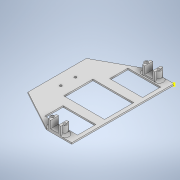
# Autodesk Inventor part: Part4
Saved by Autodesk Inventor 2020 (Build 240168000, 168)
## iProperties
Created: 2023-02-02
Part Number: Part4
Material: Generic
Document SubType Name: Modeling
Designer: aniela
Density: 1 g/cm^3
Appearance: Default
Author: aniela
Autodesk Inventor part; units mm, degrees
ref_plane "YZ Plane" through (0, 0, 0) normal (1, 0, 0) x (0, 1, 0)
ref_plane "XZ Plane" through (0, 0, 0) normal (0, 1, 0) x (-1, 0, 0)
ref_plane "XY Plane" through (0, 0, 0) normal (0, 0, 1) x (1, 0, 0)
sketch "Sketch1" plane through (0, 0, 0) normal (0, 1, 0) x (-1, 0, 0)
  line L0 (0, 0) -> (35, 0) construction
  line L1 (90, 30) -> (90, 110) construction
  line L2 (35, 140) -> (0, 140)
  line L3 (0, 140) -> (0, 0)
  line L4 (0, 0) -> (35, 0) construction
  line L5 (35, 0) -> (35, 140) construction
  line L6 (35, 140) -> (0, 140) construction
  line L7 (0, 140) -> (0, 0) construction
  line L8 (90, 110) -> (35, 140) construction
  line L9 (35, 0) -> (90, 30) construction
  line L10 (35, 140) -> (90, 110) construction
  line L11 (35, 0) -> (90, 30) construction
  line L12 (90, 110) -> (90, 30) construction
  line L13 (35, 0) -> (90, 30)
  line L14 (90, 30) -> (90, 110)
  line L15 (90, 110) -> (35, 140)
  line L16 (5, 127) -> (50, 127) construction
  line L17 (50, 127) -> (50, 102) construction
  line L18 (50, 102) -> (5, 102) construction
  line L19 (5, 102) -> (5, 127) construction
  line L20 (50, 127) -> (50, 102) construction
  line L21 (50, 102) -> (5, 102) construction
  line L22 (50, 127) -> (50, 102)
  line L23 (50, 127) -> (5, 127)
  line L24 (50, 102) -> (5, 102)
  line L25 (5, 102) -> (5, 127)
  line L26 (35, 0) -> (0, 0) construction
  line L27 (5, 13) -> (50, 13) construction
  line L28 (50, 13) -> (50, 38) construction
  line L29 (50, 38) -> (5, 38) construction
  line L30 (5, 38) -> (5, 13) construction
  line L31 (50, 38) -> (5, 38) construction
  line L32 (5, 38) -> (5, 13) construction
  line L33 (5, 13) -> (50, 13) construction
  line L34 (50, 13) -> (50, 38) construction
  line L35 (5, 13) -> (50, 13) construction
  line L36 (50, 13) -> (50, 38) construction
  line L37 (50, 38) -> (5, 38) construction
  line L38 (5, 38) -> (5, 13) construction
  line L39 (50, 38) -> (50, 13)
  line L40 (50, 13) -> (5, 13)
  line L41 (5, 13) -> (5, 38)
  line L42 (5, 38) -> (50, 38)
  line L43 (9.9818, 0) -> (0, 0) construction
  line L44 (0, 0) -> (0, 50) construction
  line L45 (0, 50) -> (9.9818, 50) construction
  line L46 (9.9818, 50) -> (9.9818, 0) construction
  line L47 (5, 50) -> (61, 50) construction
  line L48 (61, 50) -> (61, 87) construction
  line L49 (5, 87) -> (5, 50) construction
  line L50 (5, 87) -> (5, 50) construction
  line L51 (5, 50) -> (61, 50) construction
  line L52 (61, 50) -> (61, 87) construction
  line L53 (61, 87) -> (61, 50) construction
  line L54 (61, 50) -> (5, 50)
  line L55 (35, 0) -> (0, 0)
  line L56 (61, 50) -> (61, 90)
  line L57 (61, 90) -> (5, 90)
  line L58 (5, 50) -> (5, 90)
  point P0 (90, 140)
  point P1 (90, 0)
  dimension "d0" = 90
  dimension "d1" = 140
  dimension "d3" = 30
  dimension "d4" = 55
  dimension "d7" = 80
  dimension "d9" = 45
  dimension "d10" = 25
  dimension "d11" = 35
  dimension "d12" = 13
  dimension "d13" = 5
  dimension "d14" = 25
  dimension "d15" = 45
  dimension "d16" = 5
  dimension "d17" = 50
  dimension "d18" = 56
  dimension "d108" = 12
  dimension "d110" = 12
  dimension "d112" = 40
  constraints: 118 end point, 18 collinear, 16 parallel, 9 perpendicular, 9 point on line, 8 horizontal, 1 vertical
  measures "d0" distance of L2.end point (90, 140)
  measures "d1" distance of point (90, 140) point (90, 0)
  measures "d3" distance of L1.end point (90, 140)
  measures "d4" distance of L2.start point (90, 140)
  measures "d7" distance of L1.start L1.end
  measures "d9" distance of L17.end L18.end
  measures "d10" distance of L16.end L17.end
  measures "d11" distance of L2.start L2.end
  measures "d12" distance between parallel lines of L2 L16
  measures "d13" distance from line of L3 L18.end
  measures "d14" distance of L28.end L27.end
  measures "d15" distance of L28.end L31.end
  measures "d16" distance from line of L3 L27.start
  measures "d17" distance of L43.end L44.end
  measures "d18" distance of L49.start L48.end
  measures "d108" distance between parallel lines of L47 L37
  measures "d110" distance between parallel lines of L18 L57
  measures "d112" distance of L51.end L56.end
sketch "Sketch2" plane through (0, 0, 0) normal (0, 1, 0) x (-1, 0, 0)
  point P0 (0, 0)
sketch "Sketch3" plane through (0, 0, 0) normal (0, 1, 0) x (-1, 0, 0)
  point P0 (0, 0)
sketch "Sketch4" plane through (0, 0, 0) normal (0, 1, 0) x (-1, 0, 0)
  line L0 (0, 0) -> (35.5492, 0)
  line L1 (0, 0) -> (35, 0) construction
  line L2 (35, 0) -> (90, 30) construction
  line L3 (35, 0) -> (0, 0)
  constraints: 4 end point, 2 horizontal
extrude "Extrusion1" add sketch "Sketch1" along normal blind 2
sketch "Sketch5" plane through (0, 2, 0) normal (0, 1, 0) x (1, 0, 0)
  line L0 (0, 0) -> (-35, 0) projected
  line L1 (-15, 0) -> (-32, 0)
  line L2 (-32, 0) -> (-32, -11)
  line L3 (-32, -11) -> (-15, -11)
  line L4 (-15, -11) -> (-15, 0)
  line L5 (-32, 0) -> (-15, 0)
  line L6 (-15, 0) -> (-15, -11)
  line L7 (-15, -11) -> (-32, -11)
  line L8 (-32, -11) -> (-32, 0)
  line L9 (-35, -140) -> (0, -140) projected
  line L10 (-15, -140) -> (-32, -140)
  line L11 (-32, -140) -> (-32, -129)
  line L12 (-32, -129) -> (-15, -129)
  line L13 (-15, -129) -> (-15, -140)
  line L14 (-32, -129) -> (-15, -129)
  line L15 (-15, -129) -> (-15, -140)
  line L16 (-15, -140) -> (-32, -140)
  line L17 (-32, -140) -> (-32, -129)
  dimension "d22" = 17
  dimension "d23" = 11
  dimension "d24" = 11
  constraints: 32 end point, 8 parallel, 4 horizontal, 4 perpendicular, 4 point on line
  measures "d22" distance of L3.end L2.end
  measures "d23" distance of L2.end L1.end
  measures "d24" distance of L10.end L11.end
extrude "Extrusion2" add sketch "Sketch5" along normal blind 2
sketch "Sketch6" plane through (0, 4, 0) normal (0, 1, 0) x (1, 0, 0)
  line L0 (-32, 0) -> (-32, -11) projected
  line L1 (-32, 0) -> (-29, 0)
  line L2 (-29, 0) -> (-29, -11)
  line L3 (-29, -11) -> (-32, -11)
  line L4 (-32, -11) -> (-32, 0)
  line L5 (-15, -11) -> (-15, 0) projected
  line L6 (-32, -11) -> (-15, -11) projected
  line L7 (-15, 0) -> (-18, 0)
  line L8 (-18, 0) -> (-18, -11)
  line L9 (-18, -11) -> (-15, -11)
  line L10 (-15, -11) -> (-15, 0)
  line L11 (-32, -11) -> (-32, 0)
  line L12 (0, 0) -> (-35, 0) projected
  line L13 (-32, -11) -> (-15, -11)
  line L14 (-32, 0) -> (-15, 0)
  line L15 (-15, -129) -> (-15, -140) projected
  line L16 (-32, -129) -> (-15, -129) projected
  line L17 (-15, -140) -> (-18, -140)
  line L18 (-18, -140) -> (-18, -129)
  line L19 (-18, -129) -> (-15, -129)
  line L20 (-15, -129) -> (-15, -140)
  line L21 (-32, -129) -> (-29, -129)
  line L22 (-29, -129) -> (-29, -140)
  line L23 (-29, -140) -> (-32, -140)
  line L24 (-32, -140) -> (-32, -129)
  line L25 (-35, -140) -> (-32, -140) projected
  line L26 (-32, -140) -> (-32, -129)
  line L27 (-32, -129) -> (-15, -129)
  line L28 (-18, -129) -> (-18, -140)
  line L29 (-35, -140) -> (0, -140) projected
  line L30 (-29, -129) -> (-29, -140)
  dimension "d27" = 3
  dimension "d28" = 3
  constraints: 46 end point, 11 equal length, 8 perpendicular, 4 horizontal, 4 point on line
  measures "d27" distance of L2.end L3.end
  measures "d28" distance of L9.end L8.end
extrude "Extrusion3" add sketch "Sketch6" along normal blind 10 contours L15 L17 L18 L16 | L22 L23 L24 L16
sketch "Sketch7" plane through (0, 4, 0) normal (0, 1, 0) x (1, 0, 0)
  line L0 (-15, -11) -> (-15, 0) projected
  line L1 (-32, -11) -> (-15, -11) projected
  line L2 (-15, 0) -> (-18, 0)
  line L3 (-18, 0) -> (-18, -11)
  line L4 (-18, -11) -> (-15, -11)
  line L5 (-15, -11) -> (-15, 0)
  line L6 (-18, -11) -> (-15, -11)
  line L7 (-15, -11) -> (-15, 0)
  line L8 (-15, 0) -> (-18, 0)
  line L9 (-18, 0) -> (-18, -11)
  line L10 (-32, 0) -> (-32, -11) projected
  line L11 (-32, 0) -> (-29, 0)
  line L12 (-29, 0) -> (-29, -11)
  line L13 (-29, -11) -> (-32, -11)
  line L14 (-32, -11) -> (-32, 0)
  line L15 (-18, -11) -> (-29, -11)
  point P0 (0, 0)
  dimension "d31" = 3
  dimension "d32" = 3
  constraints: 26 end point, 6 parallel, 4 perpendicular, 3 horizontal, 2 point on line
  measures "d31" distance of L4.end L3.end
  measures "d32" distance of L12.end L13.end
extrude "Extrusion4" add sketch "Sketch7" along normal blind 10
sketch "Sketch8" plane through (0, 2, 0) normal (0, 1, 0) x (1, 0, 0)
  line L0 (-80, -55) -> (-70, -55)
  line L1 (-70, -55) -> (-70, -85)
  line L2 (-70, -85) -> (-80, -85)
  line L3 (-80, -85) -> (-80, -55)
  circle A0 centre (-75, -60) radius 1.5
  circle A1 centre (-75, -80) radius 1.5
  point P0 (0, 0)
  dimension "d35" = 10
  dimension "d36" = 30
  dimension "d37" = 3
  dimension "d38" = 3
  constraints: 8 end point, 2 centre point, 2 parallel, 1 horizontal, 1 perpendicular
  measures "d35" distance of L1.end L2.end
  measures "d36" distance of L0.end L1.end
  measures "d37" diameter of A0
  measures "d38" diameter of A1
extrude "Extrusion5" cut sketch "Sketch8" along normal blind 2
sketch "Sketch9" plane through (-75, 2, 80) normal (0, 1, 0) x (1, 0, 0)
  point P0 (75, 80)
  point P1 (-0.0687, 0.0063)
hole "Hole1" at (-75.0687, 2, 79.9937) direction (0, -1, 0) diameter 3 end through all
sketch "Sketch10" plane through (-75, 2, 60) normal (0, 1, 0) x (1, 0, 0)
  point P0 (75, 60)
  point P1 (-0.0342, 0.0658)
hole "Hole2" at (-75.0342, 2, 59.9342) direction (0, -1, 0) diameter 3 end through all
sketch "Sketch11" plane through (0, 14, 0) normal (0, 1, 0) x (1, 0, 0)
  line L0 (-15, 0) -> (-15, -11) projected
  circle A0 centre (-15, -5.5) radius 3
  line L1 (-32, -11) -> (-32, 0) projected
  circle A1 centre (-32, -5.5) radius 3
  point P0 (0, 0)
  point P1 (-15, -2.5)
  point P2 (-15, -8.5)
  point P3 (-32, -2.5)
  point P4 (-32, -8.5)
  dimension "d55" = 6
  dimension "d56" = 6
  constraints: 2 centre point, 2 midpoint
  measures "d55" diameter of A0
  measures "d56" diameter of A1
extrude "Extrusion6" add sketch "Sketch11" against normal blind 12 contours A0 L0 | A1 L1 picked at (-13.8765, -5.0912) picked at (-33.7524, -6.0681)
sketch "Sketch12" plane through (0, 14, 0) normal (0, 1, 0) x (1, 0, 0)
  arc A0 (-15, -8.5) -> (-15, -2.5) centre (-15, -5.5) ccw projected
  circle A1 centre (-15, -5.5) radius 2
  point P0 (0, 0)
  dimension "d59" = 4
  constraints: 1 centre point, 1 coincident
  measures "d59" diameter of A1
sketch "Sketch13" plane through (0, 14, 0) normal (0, 1, 0) x (1, 0, 0)
  arc A0 (-32, -2.5) -> (-32, -8.5) centre (-32, -5.5) ccw projected
  circle A1 centre (-32, -5.5) radius 2
  point P0 (0, 0)
  dimension "d60" = 4
  constraints: 1 centre point, 1 coincident
  measures "d60" diameter of A1
hole "Hole3" at (-32, 14, 5.5) direction (0, -1, 0) diameter 4 end through all
hole "Hole4" at (-15, 14, 5.5) direction (0, -1, 0) diameter 4 end through all
sketch "Sketch14" plane through (0, 0, 0) normal (0, -1, 0) x (1, 0, 0)
  circle A0 centre (-15, 5.5) radius 2 projected
  circle A1 centre (-15, 5.5) radius 2
  circle A2 centre (-32, 5.5) radius 2 projected
  circle A3 centre (-32, 5.5) radius 2
  circle A4 centre (-15, 5.5) radius 2
  point P0 (0, 0)
  constraints: 3 centre point, 3 coincident, 1 concentric
extrude "Extrusion7" add sketch "Sketch14" against normal blind 2
sketch "Sketch15" plane through (0, 14, 0) normal (0, 1, 0) x (1, 0, 0)
  line L0 (-15, -140) -> (-15, -129) projected
  circle A0 centre (-15, -134.5) radius 3
  line L1 (-18, -129) -> (-18, -140) projected
  point P0 (0, 0)
  constraints: 1 centre point, 1 midpoint, 1 tangent
extrude "Extrusion8" add sketch "Sketch15" against normal blind 12
sketch "Sketch16" plane through (0, 14, 0) normal (0, 1, 0) x (1, 0, 0)
  line L0 (-32, -140) -> (-32, -129) projected
  circle A0 centre (-32, -134.5) radius 3.0002
  point P0 (0, 0)
  point P1 (-32, -131.4998)
  point P2 (-32, -137.5002)
  constraints: 1 centre point, 1 midpoint
extrude "Extrusion9" add sketch "Sketch16" against normal blind 12 contours A0 L0 picked at (-33.3017, -133.9319)
sketch "Sketch17" plane through (0, 14, 0) normal (0, 1, 0) x (1, 0, 0)
  arc A0 (-15, -137.5) -> (-15, -131.5) centre (-15, -134.5) ccw projected
  circle A1 centre (-15, -134.5) radius 2
  arc A2 (-32, -131.4998) -> (-32, -137.5002) centre (-32, -134.5) ccw projected
  circle A3 centre (-32, -134.5) radius 2
  point P0 (0, 0)
  dimension "d81" = 4
  dimension "d82" = 4
  constraints: 2 centre point, 2 coincident
  measures "d81" diameter of A1
  measures "d82" diameter of A3
hole "Hole5" at (-32, 14, 134.5) direction (0, -1, 0) diameter 4 end through all
sketch "Sketch18" plane through (0, 14, 0) normal (0, 1, 0) x (1, 0, 0)
  arc A0 (-15, -137.5) -> (-15, -131.5) centre (-15, -134.5) ccw projected
  circle A1 centre (-15, -134.5) radius 2
  point P0 (0, 0)
  dimension "d7" = 80
  dimension "d11" = 35
  dimension "d90" = 4
  constraints: 1 centre point, 1 coincident
  measures "d90" diameter of A1
hole "Hole6" at (-15, 14, 134.5) direction (0, -1, 0) diameter 4 end through all
sketch "Sketch19" plane through (0, 0, 0) normal (0, -1, 0) x (1, 0, 0)
  point P0 (0, 0)
sketch "Sketch20" plane through (0, 14, 0) normal (0, 1, 0) x (1, 0, 0)
  circle A0 centre (-32, -134.5) radius 2 projected
  circle A1 centre (-32, -134.5) radius 2
  circle A2 centre (-15, -134.5) radius 2 projected
  circle A3 centre (-15, -134.5) radius 2
  point P0 (0, 0)
  constraints: 2 centre point, 2 coincident
extrude "Extrusion10" add sketch "Sketch20" against normal up to surface (14 mm away)
sketch "Sketch21" plane through (0, 0, 0) normal (0, -1, 0) x (1, 0, 0)
  point P0 (0, 0)
sketch "Sketch22" plane through (0, 14, 0) normal (0, 1, 0) x (1, 0, 0)
  arc A0 (-15, -137.5) -> (-15, -131.5) centre (-15, -134.5) ccw projected
  circle A1 centre (-15, -134.5) radius 2
  arc A2 (-32, -131.4998) -> (-32, -137.5002) centre (-32, -134.5) ccw projected
  circle A3 centre (-32, -134.5) radius 2
  point P0 (0, 0)
  dimension "d100" = 4
  dimension "d101" = 4
  constraints: 2 centre point, 2 coincident
  measures "d100" diameter of A1
  measures "d101" diameter of A3
extrude "Extrusion11" cut sketch "Sketch22" against normal blind 12 contours A1
sketch "Sketch23" plane through (0, 14, 0) normal (0, 1, 0) x (1, 0, 0)
  arc A0 (-32, -131.4998) -> (-32, -137.5002) centre (-32, -134.5) ccw projected
  circle A1 centre (-32, -134.5) radius 2
  point P0 (0, 0)
  dimension "d104" = 4
  constraints: 1 centre point, 1 coincident
  measures "d104" diameter of A1
extrude "Extrusion12" cut sketch "Sketch23" against normal blind 12
sketch "Sketch24" plane through (0, 2, 0) normal (0, 1, 0) x (1, 0, 0)
  point P0 (0, 0)
fillet "Fillet1" radius 3 1 edges at (-35, 2, 5.5)
fillet "Fillet2" radius 3 1 edges at (-12, 2, 5.5)
fillet "Fillet3" radius 3 1 edges at (-12, 2, 134.5)
fillet "Fillet4" radius 3 1 edges at (-35.0002, 2, 134.5)
body "Solid1"
